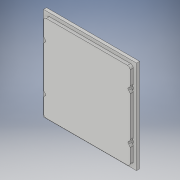
# Autodesk Inventor part: Lid
Saved by Autodesk Inventor 2018 (Build 220112000, 112)
## iProperties
Created: 2018-04-20
Part Number: Lid
Material: Generic
Document SubType Name: Modeling
Designer: MIABo
Density: 1 g/cm^3
Appearance: Default
Author: MIABo
Autodesk Inventor part; units mm, degrees
ref_plane "YZ Plane" through (0, 0, 0) normal (1, 0, 0) x (0, 1, 0)
ref_plane "XZ Plane" through (0, 0, 0) normal (0, 1, 0) x (-1, 0, 0)
ref_plane "XY Plane" through (0, 0, 0) normal (0, 0, 1) x (1, 0, 0)
sketch "Sketch1" plane through (0, 0, 0) normal (0, 0, 1) x (1, 0, 0)
  line L0 (0, 0) -> (-114.3, 0)
  line L1 (-114.3, 0) -> (-114.3, 114.3)
  line L2 (-114.3, 114.3) -> (0, 114.3)
  line L3 (0, 114.3) -> (0, 0)
  line L4 (-3.81, 3.81) -> (-110.49, 3.81)
  line L5 (-110.49, 3.81) -> (-110.49, 110.49)
  line L6 (-110.49, 110.49) -> (-3.81, 110.49)
  line L7 (-3.81, 110.49) -> (-3.81, 3.81)
  dimension "d0" = 3.81
  dimension "d1" = 3.81
  dimension "d2" = 3.81
  dimension "d3" = 3.81
  dimension "d4" = 114.3
  dimension "d5" = 114.3
  constraints: 16 end point, 4 parallel, 2 horizontal, 2 perpendicular, 1 coincident
  measures "d0" distance between parallel lines of L3 L7
  measures "d1" distance between parallel lines of L1 L5
  measures "d2" distance between parallel lines of L2 L6
  measures "d3" distance between parallel lines of L0 L4
  measures "d4" distance of L1.end L2.end
  measures "d5" distance of L0.end L1.end
extrude "Extrusion1" add sketch "Sketch1" along normal blind 3.81 contours L0 L1 L2 L3 | L4 L5 L6 L7
sketch "Sketch2" plane through (0, 0, 3.81) normal (0, 0, 1) x (1, 0, 0)
  line L0 (-4.064, 4.064) -> (-110.236, 4.064)
  line L1 (-110.236, 4.064) -> (-110.236, 110.236)
  line L2 (-110.236, 110.236) -> (-4.064, 110.236)
  line L3 (-4.064, 110.236) -> (-4.064, 4.064)
  line L4 (-114.3, 114.3) -> (-114.3, 0) projected
  line L5 (0, 114.3) -> (-114.3, 114.3) projected
  line L6 (0, 0) -> (0, 114.3) projected
  line L7 (-114.3, 0) -> (0, 0) projected
  dimension "d8" = 4.064
  dimension "d9" = 4.064
  dimension "d10" = 4.064
  dimension "d11" = 4.064
  constraints: 8 end point, 2 parallel, 1 horizontal, 1 perpendicular
  measures "d8" distance between parallel lines of L4 L1
  measures "d9" distance between parallel lines of L5 L2
  measures "d10" distance between parallel lines of L6 L3
  measures "d11" distance between parallel lines of L7 L0
extrude "Extrusion2" add sketch "Sketch2" along normal blind 3.81 contours L0 L1 L2 L3
fillet "Fillet1" radius 3.175 4 edges at (-4.064, 110.236, 5.715) (-110.236, 110.236, 5.715) (-110.236, 4.064, 5.715) (-4.064, 4.064, 5.715)
sketch "Sketch3" plane through (0, 0, 0) normal (0, 0, -1) x (-1, 0, 0)
  circle A0 centre (109.22, 85.725) radius 1.651
  circle A1 centre (109.22, 28.575) radius 1.651
  line L0 (114.3, 0) -> (114.3, 114.3)
  line L1 (114.3, 114.3) -> (0, 114.3)
  circle A2 centre (5.08, 85.725) radius 1.651
  circle A3 centre (5.08, 28.575) radius 1.651
  line L2 (0, 114.3) -> (0, 0)
  line L3 (0, 0) -> (114.3, 0)
  dimension "d15" = 3.302
  dimension "d16" = 57.15
  dimension "d17" = 57.15
  dimension "d18" = 104.14
  dimension "d19" = 104.14
  dimension "d20" = 28.575
  dimension "d21" = 114.3
  dimension "d22" = 5.08
  dimension "d23" = 5.08
  dimension "d24" = 5.08
  dimension "d37" = 114.3
  dimension "d38" = 114.3
  dimension "d39" = 114.3
  dimension "d40" = 114.3
  constraints: 8 end point, 4 centre point, 3 equal radius, 2 parallel, 1 horizontal, 1 vertical
  measures "d15" diameter of A0
  measures "d16" distance of A3.centre A2.centre
  measures "d17" distance of A1.centre A0.centre
  measures "d18" distance of A2.centre A0.centre
  measures "d19" distance of A3.centre A1.centre
  measures "d20" distance from line of L1 A0.centre
  measures "d21" distance of L0.start L0.end
  measures "d22" distance from line of A0.centre L0
  measures "d23" distance from line of L2 A3.centre
  measures "d24" distance from line of L0 A1.centre
  measures "d37" distance between parallel lines of L3 L1
  measures "d38" distance between parallel lines of L2 L0
  measures "d39" distance from line of point (0, 0) L1
  measures "d40" distance from line of point (0, 0) L0
extrude "Extrusion3" cut sketch "Sketch3" against normal up to surface (7.62 mm away) contours A0 | A1 | A2 | A3
fillet "Fillet2" radius 3.175 8 edges at (-4.064, 27.2736, 5.715) (-4.064, 29.8764, 5.715) (-4.064, 84.4236, 5.715) (-4.064, 87.0264, 5.715) (-110.236, 87.0264, 5.715) (-110.236, 84.4236, 5.715) (-110.236, 29.8764, 5.715) (-110.236, 27.2736, 5.715)
equation "\"d1\" = d0"
equation "\"d2\" = d0"
equation "\"d3\" = d0"
equation "\"d16\" = d17"
equation "\"d19\" = d18"
equation "\"d23\" = d22"
equation "\"d24\" = d22"
body "Solid1"
